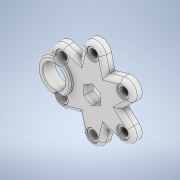
# Autodesk Inventor part: GenevaDrive3
Saved by Autodesk Inventor 2020.1 (Build 241239000, 239)
## iProperties
Created: 2019-11-09
Part Number: GenevaDrive3
Material: ABS Plastic
Document SubType Name: Modeling
Designer: Paul Lefeuvre
Density: 1.06 g/cm^3
Appearance: Smooth - White
Author: Paul Lefeuvre
Autodesk Inventor part; units mm, degrees
ref_plane "YZ Plane" through (0, 0, 0) normal (1, 0, 0) x (0, 1, 0)
ref_plane "XZ Plane" through (0, 0, 0) normal (0, 1, 0) x (-1, 0, 0)
ref_plane "XY Plane" through (0, 0, 0) normal (0, 0, 1) x (1, 0, 0)
sketch "Sketch1" plane through (0, 0, 0) normal (0, 0, 1) x (1, 0, 0)
  line L0 (0, 7.3323) -> (6.35, 3.6662) construction
  line L1 (6.35, 3.6662) -> (6.35, -3.6662) construction
  line L2 (6.35, -3.6662) -> (0, -7.3323) construction
  line L3 (0, -7.3323) -> (-6.35, -3.6662) construction
  line L4 (-6.35, -3.6662) -> (-6.35, 3.6662) construction
  line L5 (-6.35, 3.6662) -> (0, 7.3323) construction
  line L6 (6.75, 3.8971) -> (0, 7.7942)
  line L7 (0, 7.7942) -> (-6.75, 3.8971)
  line L8 (-6.75, 3.8971) -> (-6.75, -3.8971)
  line L9 (-6.75, -3.8971) -> (0, -7.7942)
  line L10 (0, -7.7942) -> (6.75, -3.8971)
  line L11 (6.75, -3.8971) -> (6.75, 3.8971)
  circle A0 centre (0, 0) radius 28.541 construction
  circle A1 centre (0, 28.541) radius 3.3
  circle A2 centre (-28.541, 0) radius 8.5 construction
  circle A3 centre (-28.541, 0) radius 9.1
  circle A4 centre (0, 28.541) radius 4.75
  line L12 (8.0146, 30.5055) -> (10.875, 18.8361)
  line L13 (0, 0) -> (19.7475, 34.2037) construction
  line L14 (-8.0146, 30.5055) -> (-10.875, 18.8361)
  arc A5 (8.0146, 30.5055) -> (-8.0146, 30.5055) centre (0, 28.541) ccw
  line L15 (0, 0) -> (0, 36.7928) construction
  line L16 (10.875, 18.8361) -> (3.375, 5.8457)
  line L17 (-3.375, 5.8457) -> (-10.875, 18.8361)
  line L18 (0, 0) -> (-55.6382, 0) construction
  circle A6 centre (-24.7172, -14.2705) radius 3.3
  circle A7 centre (-24.7172, -14.2705) radius 4.75
  circle A8 centre (-24.7172, 14.2705) radius 3.3
  circle A9 centre (-24.7172, 14.2705) radius 4.75
  arc A10 (-21.3322, -10.9382) -> (-21.3322, 10.9382) centre (-28.541, 0) ccw
  arc A11 (-29.3149, 13.0771) -> (-29.3149, -13.0771) centre (-28.541, 0) ccw
  arc A12 (-26.7417, 9.9735) -> (-26.7417, -9.9735) centre (0, 0) ccw
  dimension "d0" = 12.7
  dimension "d1" = 0.4
  dimension "d3" = 6.6
  dimension "d9" = 17
  dimension "d10" = 0.6
  dimension "d14" = 9.5
  dimension "d31" = 30
  dimension "d58" = 57.082
  dimension "d59" = 6.6
  dimension "d60" = 9.5
  dimension "d61" = 6.6
  dimension "d62" = 9.5
  constraints: 38 end point, 19 point on circle, 13 centre point, 6 coincident, 4 point on line, 2 midpoint, 2 tangent, 1 horizontal, 1 perpendicular, 1 vertical, 18 other
  measures "d0" distance of L4.end L0.end
  measures "d1" distance between parallel lines of L0 L6
  measures "d3" diameter of A1
  measures "d9" diameter of A2
  measures "d10" radial gap between concentric circles of A2 A3
  measures "d14" diameter of A4
  measures "d31" angle of L15 L13
  measures "d58" diameter of A0
  measures "d59" diameter of A6
  measures "d60" diameter of A7
  measures "d61" diameter of A8
  measures "d62" diameter of A9
extrude "Extrusion1" add sketch "Sketch1" along normal blind 7.5 contours L6 L7 L17 L14 A5 L12 L16
fillet "Fillet1" radius 3.45 3 edges at (-9.4448, 24.6708, 7.5) (9.4448, 24.6708, 7.5) (0, 36.7928, 7.5)
extrude "Extrusion2" add sketch "Sketch1" along normal blind 6.5 contours A4
fillet "Fillet3" radius 0.5 1 edges at (-4.75, 28.541, 7.5)
pattern_circular "Circular Pattern1" count 6 over 360 about axis through (0, 0, 0) along (0, 0, -1) of "Extrusion1", "Fillet1", "Fillet3", "Extrusion2"
extrude "Extrusion3" cut sketch "Sketch1" along normal blind 10 contours A3 A12 | A12 A3
extrude "Extrusion4" add sketch "Sketch1" along normal blind 10 contours A3 A12 A9 A10 A7 | A3 A12 A7 A11 A9
fillet "Fillet7" radius 0.5 1 edges at (-37.641, 0, 10)
fillet "Fillet8" radius 1 2 edges at (-41.641, 0, 10) (-15.441, 0, 10)
body "Solid1"
